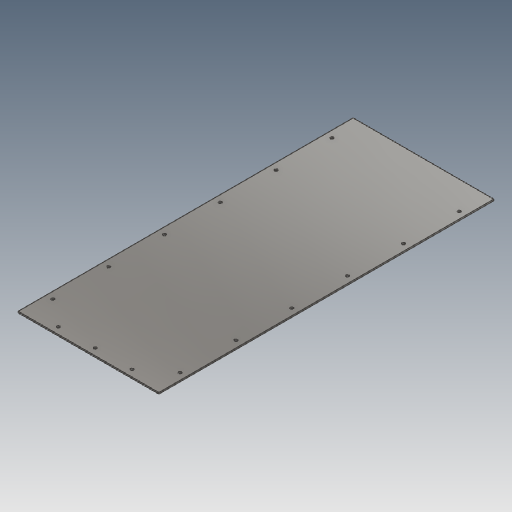
# Autodesk Inventor part: 100-10-FRAME-BOTTOM-PLATE
Saved by Autodesk Inventor 2018.2 (Build 222227000, 227)
## iProperties
Manager: feesmrt
Company: FRANCOR
Part Number: 100-10-FRAME-BOTTOM-PLATE
Material: Edelstahl
Document SubType Name: Modeling
Designer: feesmrt
Density: 8 g/cm^3
Appearance: Halbpoliert
Project: Rescue Robot
Cost Center: -
Engineer: feesmrt
Authority: feesmrt
Description: Chassis Frame Bottom Plate
Stock Number: 100-10-FRAME-BOTTOM-PLATE
Author: feesmrt
Subject: Rescue Robot
Revision Number: 1
Title: Chassis Frame Bottom Plate
Autodesk Inventor part; units mm, degrees
ref_plane "YZ Plane" through (0, 0, 0) normal (1, 0, 0) x (0, 1, 0)
ref_plane "XZ Plane" through (0, 0, 0) normal (0, 1, 0) x (-1, 0, 0)
ref_plane "XY Plane" through (0, 0, 0) normal (0, 0, 1) x (1, 0, 0)
sketch "Skizze1" plane through (0, 0, 0) normal (0, 0, 1) x (1, 0, 0)
  line L0 (-105, -250) -> (105, -250)
  line L1 (105, -250) -> (105, 250)
  line L2 (105, 250) -> (-105, 250)
  line L3 (-105, 250) -> (-105, -250)
  line L4 (-105, -250) -> (105, 250) construction
  line L5 (105, -250) -> (-105, 250) construction
  point P0 (0, 0)
  dimension "d0" = 500
  dimension "d1" = 210
  constraints: 12 end point, 2 midpoint, 2 parallel, 1 horizontal, 1 perpendicular
  measures "d0" distance of L0.end L1.end
  measures "d1" distance of L1.end L2.end
extrude "Grundkörper" add sketch "Skizze1" along normal mid plane 2
sketch "Skizze2" plane through (0, 0, 1) normal (0, 0, 1) x (1, 0, 0)
  line L0 (-105, 250) -> (-105, -250) construction
  line L1 (0, 350) -> (0, -350) construction
  line L2 (-147, 0) -> (147, 0) construction
  line L3 (105, 250) -> (-105, 250) construction
  line L4 (-95, 250) -> (-95, -250) construction
  line L5 (-105, -250) -> (105, -250) construction
  line L6 (-95, -240) -> (105, -240) construction
  line L7 (105, -250) -> (105, 250) construction
  point P0 (0, 0)
  point P1 (-95, -208.3333)
  point P2 (-95, -125)
  point P3 (-95, -41.6667)
  point P4 (-95, 41.6667)
  point P5 (-95, 125)
  point P6 (-95, 208.3333)
  point P7 (95, -208.3333)
  point P8 (95, -125)
  point P9 (95, -41.6667)
  point P10 (95, 41.6667)
  point P11 (95, 125)
  point P12 (95, 208.3333)
  point P13 (0, -240)
  point P14 (55, -240)
  point P15 (-55, -240)
  dimension "d4" = 10
  dimension "d20" = 41.6667
  dimension "d23" = 83.3333
  dimension "d28" = 10
  dimension "d29" = 110
  constraints: 9 point on line, 7 symmetric about line, 4 end point, 1 horizontal, 1 perpendicular, 1 vertical, 5 other
  measures "d4" distance between parallel lines of L0 L4
  measures "d20" distance from line of point (-95, -208.333) L5
  measures "d23" distance of point (-95, -208.333) point (-95, -125)
  measures "d28" distance between parallel lines of L5 L6
  measures "d29" distance of point (-55, -240) point (55, -240)
hole "M4_Boh" at (-95, -208.3333, 1) at (-95, -125, 1) at (-95, -41.6667, 1) at (-95, 41.6667, 1) at (-95, 125, 1) at (-95, 208.3333, 1) at (95, 208.3333, 1) at (95, 125, 1) at (95, 41.6667, 1) at (95, -41.6667, 1) at (95, -125, 1) at (95, -208.3333, 1) at (-55, -240, 1) at (0, -240, 1) at (55, -240, 1) direction (0, 0, -1) diameter 4.5 end through all
equation "\"d0\" = Chassis_Length"
equation "\"d20\" = 0.0833333 * Chassis_Length"
equation "\"d23\" = 0.166667 * Chassis_Length"
equation "\"d28\" = d4"
equation "\"d29\" = 0.5 * Chassis_Width"
equation "\"Chassis_Length\" = 500"
equation "\"Rocker_Screw_Distance\" = 32.5"
equation "\"Rocker_Screw_Distance_Bottom\" = 76"
equation "\"Chassis_Width\" = 220"
